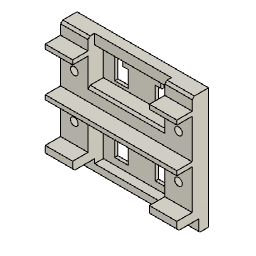
スタンドカップラー v1 (Autodesk Fusion 360 design; units mm, degrees)
Autodesk Fusion 360 part; units mm, degrees
note: some values were not read from the file. Chosen so that the rebuilt part matches the saved one: which bodies a step acts on; which face or edge a step refers to. Set by a fixed rule: which sketch regions a step uses.
sketch "スケッチ1" plane through (0, 0, 0) normal (0, 1, 0) x (1, 0, 0)
  line L0 (12.35, 21.95) -> (-12.35, 21.95) construction
  line L1 (-12.35, 21.95) -> (-12.35, -21.95) construction
  line L2 (-12.35, -21.95) -> (12.35, -21.95) construction
  line L3 (12.35, -21.95) -> (12.35, 21.95) construction
  line L4 (12.35, 21.95) -> (-12.35, -21.95) construction
  line L5 (-12.35, 21.95) -> (12.35, -21.95) construction
  line L6 (12.35, -21.95) -> (8.65, -21.95)
  line L7 (8.65, -21.95) -> (8.65, -15.35)
  line L8 (8.65, -8.35) -> (12.35, -8.35)
  line L9 (12.35, -8.35) -> (12.35, -21.95)
  line L10 (12.35, -8.35) -> (6.15, -8.35)
  line L11 (6.15, -8.35) -> (6.15, -15.35)
  line L12 (6.15, -15.35) -> (8.65, -15.35)
  line L13 (12.35, -15.35) -> (12.35, -8.35)
  line L14 (12.35, 21.95) -> (12.35, 8.35)
  line L15 (12.35, 14.95) -> (12.35, 21.95)
  line L16 (8.65, 21.95) -> (12.35, 21.95)
  line L17 (12.35, 21.95) -> (6.15, 21.95)
  line L18 (12.35, 8.35) -> (8.65, 8.35)
  line L19 (8.65, 8.35) -> (8.65, 14.95)
  line L20 (6.15, 14.95) -> (8.65, 14.95)
  line L21 (6.15, 21.95) -> (6.15, 14.95)
  line L22 (0, 0) -> (0, -7)
  line L23 (-12.35, 21.95) -> (12.35, 21.95) construction
  line L24 (-12.35, -8.35) -> (-12.35, -21.95)
  line L25 (-6.15, -15.35) -> (-8.65, -15.35)
  line L26 (-12.35, -21.95) -> (-8.65, -21.95)
  line L27 (-8.65, -21.95) -> (-8.65, -15.35)
  line L28 (-12.35, 21.95) -> (-6.15, 21.95)
  line L29 (-12.35, 21.95) -> (12.35, -21.95) construction
  line L30 (-12.35, -21.95) -> (-12.35, 21.95) construction
  line L31 (-8.65, 21.95) -> (-12.35, 21.95)
  line L32 (-8.65, 8.35) -> (-8.65, 14.95)
  line L33 (12.35, 21.95) -> (-12.35, -21.95) construction
  line L34 (12.35, -21.95) -> (-12.35, -21.95) construction
  line L35 (-12.35, 8.35) -> (-8.65, 8.35)
  line L36 (-6.15, 21.95) -> (-6.15, 14.95)
  line L37 (-8.65, -8.35) -> (-12.35, -8.35)
  line L38 (-12.35, -15.35) -> (-12.35, -8.35)
  line L39 (-6.15, 14.95) -> (-8.65, 14.95)
  line L40 (-6.15, -8.35) -> (-6.15, -15.35)
  line L41 (-12.35, 21.95) -> (-12.35, 8.35)
  line L42 (-12.35, -8.35) -> (-6.15, -8.35)
  line L43 (-12.35, 14.95) -> (-12.35, 21.95)
  line L44 (22.5, 32.5) -> (-22.5, 32.5)
  line L45 (-22.5, 32.5) -> (-22.5, -32.5)
  line L46 (-22.5, -32.5) -> (22.5, -32.5)
  line L47 (22.5, -32.5) -> (22.5, 32.5)
  line L48 (22.5, 32.5) -> (-22.5, -32.5) construction
  line L49 (-22.5, 32.5) -> (22.5, -32.5) construction
  dimension "d1" = 24.7
  dimension "d2" = 43.9
  dimension "d3" = 3.7
  dimension "d4" = 13.6
  dimension "d5" = 6.2
  dimension "d6" = 7
  dimension "d7" = 3.7
  dimension "d8" = 13.6
  dimension "d9" = 6.2
  dimension "d10" = 7
  dimension "d11" = 45
  dimension "d12" = 65
  constraint horizontal L0
  constraint perpendicular L0 L1
  constraint parallel L0 L2
  constraint parallel L1 L3
  constraint coincident L4 L22.start
  constraint coincident L5 L22.start
  constraint coincident L22.start origin
  constraint horizontal L6
  constraint vertical L7
  constraint horizontal L8
  constraint vertical L9
  constraint horizontal L10
  constraint vertical L11
  constraint horizontal L12
  constraint vertical L13
  constraint horizontal L18
  constraint vertical L19
  constraint horizontal L16
  constraint vertical L14
  constraint horizontal L17
  constraint vertical L21
  constraint horizontal L20
  constraint vertical L15
  constraint vertical L22
  constraint symmetric L0.start L22 L0.end
  constraint symmetric L0.end L22 L0.start
  constraint symmetric L1.end L22 L2.end
  constraint symmetric L2.end L22 L1.end
  constraint symmetric L6.end L22 L26.end
  constraint symmetric L8.start L22 L37.start
  constraint symmetric L8.end L22 L24.start
  constraint symmetric L10.end L22 L40.start
  constraint symmetric L11.end L22 L25.start
  constraint symmetric L13.start L22 L38.start
  constraint symmetric L7.end L22 L25.end
  constraint symmetric L19.end L22 L32.end
  constraint symmetric L17.end L22 L28.end
  constraint symmetric L15.start L22 L43.start
  constraint symmetric L20.start L22 L36.end
  constraint symmetric L18.end L22 L32.start
  constraint symmetric L14.end L22 L35.start
  constraint symmetric L16.start L22 L31.start
  constraint horizontal L44
  constraint perpendicular L44 L45
  constraint parallel L44 L46
  constraint parallel L45 L47
  constraint coincident L48 L22.start
  constraint coincident L49 L22.start
  measures "d1" distance of L1.end L2.end
  measures "d2" distance of L0.end L1.end
  measures "d3" distance of L2.end L6.end
  measures "d4" distance of L2.end L8.end
  measures "d5" distance of L8.end L10.end
  measures "d6" distance of L8.end L13.start
  measures "d7" distance of L18.end L14.end
  measures "d8" distance of L0.start L14.end
  measures "d9" distance of L17.end L0.start
  measures "d10" distance of L15.start L0.start
  measures "d11" distance of L45.end L46.end
  measures "d12" distance of L44.end L45.end
extrude "押し出し1" add sketch "スケッチ1" along normal blind 1.46 makes body 1
sketch "スケッチ2" plane through (0, 0, 0) normal (0, -1, 0) x (1, 0, 0)
  line L0 (12.35, -8.35) -> (12.35, -21.95)
  line L1 (12.35, -21.95) -> (6.15, -21.95)
  line L2 (6.15, -21.95) -> (6.15, -14.95)
  line L3 (6.15, -14.95) -> (8.65, -14.95)
  line L4 (8.65, -14.95) -> (8.65, -8.35)
  line L5 (8.65, -8.35) -> (12.35, -8.35)
  line L6 (-12.35, 8.35) -> (-12.35, 21.95)
  line L7 (-12.35, 21.95) -> (-8.65, 21.95)
  line L8 (-8.65, 21.95) -> (-8.65, 15.35)
  line L9 (-8.65, 15.35) -> (-6.15, 15.35)
  line L10 (-6.15, 15.35) -> (-6.15, 8.35)
  line L11 (-6.15, 8.35) -> (-12.35, 8.35)
  line L12 (-12.35, -8.35) -> (-8.65, -8.35)
  line L13 (-8.65, -8.35) -> (-8.65, -14.95)
  line L14 (-8.65, -14.95) -> (-6.15, -14.95)
  line L15 (-6.15, -14.95) -> (-6.15, -21.95)
  line L16 (-6.15, -21.95) -> (-12.35, -21.95)
  line L17 (-12.35, -21.95) -> (-12.35, -8.35)
  line L18 (12.35, 21.95) -> (12.35, 8.35)
  line L19 (12.35, 8.35) -> (6.15, 8.35)
  line L20 (6.15, 8.35) -> (6.15, 15.35)
  line L21 (6.15, 15.35) -> (8.65, 15.35)
  line L22 (8.65, 15.35) -> (8.65, 21.95)
  line L23 (8.65, 21.95) -> (12.35, 21.95)
  line L24 (22.5, -32.5) -> (22.5, 32.5)
  line L25 (22.5, 32.5) -> (-22.5, 32.5)
  line L26 (-22.5, 32.5) -> (-22.5, -32.5)
  line L27 (-22.5, -32.5) -> (22.5, -32.5)
  line L28 (-8.65, 21.95) -> (22.5, 21.95)
  line L29 (-12.35, 21.95) -> (-22.5, 21.95)
  line L30 (-12.35, -8.35) -> (-22.5, -8.35)
  line L31 (-8.65, -8.35) -> (8.65, -8.35)
  line L32 (12.35, -8.35) -> (22.5, -8.35)
  line L33 (-22.5, 0) -> (22.5, 0)
  line L34 (-6.15, 15.35) -> (6.15, 15.35)
  line L35 (-6.15, -14.95) -> (6.15, -14.95)
  constraint coincident L7.end L8.start
  constraint coincident L24 L28.end
  constraint perpendicular L24 L28
  constraint coincident L6.end L7.start
  constraint coincident L26 L29.end
  constraint perpendicular L26 L29
  constraint coincident L12.start L17.end
  constraint coincident L26 L30.end
  constraint perpendicular L26 L30
  constraint coincident L12.end L13.start
  constraint coincident L4.end L5.start
  constraint coincident L0.start L5.end
  constraint coincident L24 L32.end
  constraint perpendicular L24 L32
  constraint midpoint L26 L33.start
  constraint perpendicular L26 L33
  constraint coincident L9.end L10.start
  constraint coincident L20.end L21.start
  constraint coincident L14.end L15.start
  constraint coincident L2.end L3.start
extrude "押し出し2" add sketch "スケッチ2" along normal blind 4 contours L5 L12 L24 L26 L30 L31 L32 L33 | L3 L4 L13 L14 L31 L35 | L7 L23 L24 L25 L26 L28 L29 | L8 L9 L21 L22 L28 L34 bodies 1
move_face "面を移動1" by (0, 0, 7) 1 faces at (-7.5, -1.3333, 0) on bodies 1
sketch "スケッチ3" plane through (0, 0, 0) normal (0, -1, 0) x (1, 0, 0)
  line L0 (6.15, -14.95) -> (-6.15, -14.95)
  line L1 (-6.15, -14.95) -> (-6.15, -21.95)
  line L2 (-6.15, -21.95) -> (-12.35, -21.95)
  line L3 (-12.35, -21.95) -> (-12.35, -8.35)
  line L4 (-12.35, -8.35) -> (-22.5, -8.35)
  line L5 (-22.5, -8.35) -> (-22.5, -32.5)
  line L6 (-22.5, -32.5) -> (22.5, -32.5)
  line L7 (22.5, -32.5) -> (22.5, -8.35)
  line L8 (22.5, -8.35) -> (12.35, -8.35)
  line L9 (12.35, -8.35) -> (12.35, -21.95)
  line L10 (12.35, -21.95) -> (6.15, -21.95)
  line L11 (6.15, -21.95) -> (6.15, -14.95)
  line L12 (-22.5, -24.9494) -> (22.5, -24.9494)
  constraint coincident L5 L12.start
  constraint coincident L7 L12.end
  constraint perpendicular L7 L12
extrude "押し出し3" add sketch "スケッチ3" along normal blind 4 contours L5 L6 L7 L12 bodies 1
split "分割1" by plane through (0, 0, 0) normal (0, -1, 0) bodies 1 makes body 2 at (2.8833, -4, 1.8833) makes body 3 at (-7.5, -4, -27.4663) makes body 4 at (2.8833, -4, 28.9833)
move_face "面を移動2" by (0, 0, 6.5) 1 faces at (2.05, -2.6667, 15.35) on bodies 4
delete_face "面を削除1" 3 faces at (8.65, -2.6667, 21.9167) (2.8833, -2.6667, 21.85) (-8.65, -2.6667, 21.9167) on bodies 4
delete_face "面を削除2" 3 faces at (8.65, -1.3333, -12.75) (2.05, -2.6667, -14.95) (-8.65, -1.3333, -12.75) on bodies 2
chamfer "面取り1" distance 0.5 angle 45 1 edges at (-7.4, 0, 15.35) on bodies 1
chamfer "面取り2" distance 0.5 angle 45 3 edges at (7.4, 0, 15.35) (-7.4, 0, -14.95) (7.4, 0, -14.95) on bodies 1
sketch "スケッチ4" plane through (0, -4, 0) normal (0, -1, 0) x (1, 0, 0)
  line L0 (-22.5, -8.35) -> (22.5, -8.35)
  line L1 (22.5, -8.35) -> (22.5, 7)
  line L2 (22.5, 7) -> (-22.5, 7)
  line L3 (-22.5, 7) -> (-22.5, -8.35)
  line L4 (30, 17) -> (-30, 17)
  line L5 (-30, 17) -> (-30, -17)
  line L6 (-30, -17) -> (30, -17)
  line L7 (30, -17) -> (30, 17)
  line L8 (30, 17) -> (-30, -17) construction
  line L9 (-30, 17) -> (30, -17) construction
  line L10 (17.5, -17.4093) -> (-17.5, -17.4093)
  line L11 (-17.5, -17.4093) -> (-17.5, 17.4093)
  line L12 (-17.5, 17.4093) -> (17.5, 17.4093)
  line L13 (17.5, 17.4093) -> (17.5, -17.4093)
  line L14 (17.5, -17.4093) -> (-17.5, 17.4093) construction
  line L15 (-17.5, -17.4093) -> (17.5, 17.4093) construction
  dimension "d21" = 60
  dimension "d22" = 34
  dimension "d23" = 35
  constraint horizontal L4
  constraint perpendicular L4 L5
  constraint parallel L4 L6
  constraint parallel L5 L7
  constraint coincident L8 origin
  constraint coincident L9 origin
  constraint horizontal L10
  constraint perpendicular L10 L11
  constraint parallel L10 L12
  constraint parallel L11 L13
  constraint coincident L14 origin
  constraint coincident L15 origin
  measures "d21" distance of L5.end L6.end
  measures "d22" distance of L4.end L5.end
  measures "d23" distance of L11.end L12.end
extrude "押し出し4" add sketch "スケッチ4" against normal blind 5.46 contours L0 L2 L3 L4 L5 L6 L11 | L0 L1 L2 L4 L6 L7 L13 bodies 1 2
move_face "面を移動3" by (0, -3, 0) 1 faces at (5.8333, -4, 1.8833) on bodies 1
move_face "面を移動4" by (0, 0, -15.5) 2 faces at (-23.3333, -4.6667, -17) (23.3333, -4.6667, -17) on bodies 1
move_face "面を移動5" by (0, 0, 15.5) 2 faces at (23.3333, -4.6667, 17) (-23.3333, -4.6667, 17) on bodies 1
sketch "スケッチ5" plane through (0, -7, 0) normal (0, -1, 0) x (1, 0, 0)
  line L0 (-17.5, -8.35) -> (17.5, -8.35)
  line L1 (17.5, -8.35) -> (17.5, -32.5)
  line L2 (17.5, -32.5) -> (30, -32.5)
  line L3 (30, -32.5) -> (30, 32.5)
  line L4 (30, 32.5) -> (17.5, 32.5)
  line L5 (17.5, 32.5) -> (17.5, 7)
  line L6 (17.5, 7) -> (-17.5, 7)
  line L7 (-17.5, 7) -> (-17.5, 32.5)
  line L8 (-17.5, 32.5) -> (-30, 32.5)
  line L9 (-30, 32.5) -> (-30, -32.5)
  line L10 (-30, -32.5) -> (-17.5, -32.5)
  line L11 (-17.5, -32.5) -> (-17.5, -8.35)
  line L12 (30, -1) -> (-30, -1)
  line L13 (-30, -1) -> (-30, 1)
  line L14 (-30, 1) -> (30, 1)
  line L15 (30, 1) -> (30, -1)
  line L16 (30, -1) -> (-30, 1) construction
  line L17 (-30, -1) -> (30, 1) construction
  dimension "d26" = 60
  dimension "d27" = 2
  constraint horizontal L12
  constraint perpendicular L12 L13
  constraint parallel L12 L14
  constraint parallel L13 L15
  constraint coincident L16 origin
  constraint coincident L17 origin
  measures "d26" distance of L13.end L14.end
  measures "d27" distance of L12.end L13.end
extrude "押し出し5" add sketch "スケッチ5" along normal blind 5 contours L3 L9 L12 L13 L14 L15 bodies 1
sketch "スケッチ6" plane through (0, -7, 0) normal (0, -1, 0) x (1, 0, 0)
  line L0 (-30, 1) -> (30, 1)
  line L1 (30, 1) -> (30, 32.5)
  line L2 (30, 32.5) -> (17.5, 32.5)
  line L3 (17.5, 32.5) -> (17.5, 7)
  line L4 (17.5, 7) -> (-17.5, 7)
  line L5 (-17.5, 7) -> (-17.5, 32.5)
  line L6 (-17.5, 32.5) -> (-30, 32.5)
  line L7 (-30, 32.5) -> (-30, 1)
  line L8 (-30, 1) -> (30, 1)
  line L9 (30, 1) -> (30, 19)
  line L10 (30, 19) -> (-30, 19)
  line L11 (-30, 19) -> (-30, 1)
  line L12 (-17.5, 7) -> (-17.5, 1)
  line L13 (17.5, 7) -> (17.5, 1)
  line L14 (-6, 0) -> (5, 0)
  line L15 (30, -19) -> (-30, -19)
  line L16 (-30, -19) -> (-30, -1)
  line L17 (-17.5, -7) -> (-17.5, -32.5)
  line L18 (-17.5, -7) -> (-17.5, -1)
  line L19 (17.5, -32.5) -> (17.5, -7)
  line L20 (17.5, -7) -> (17.5, -1)
  line L21 (30, -1) -> (30, -19)
  line L22 (-30, 19) -> (30, 19)
  line L23 (30, 19) -> (30, 21)
  line L24 (30, 21) -> (-30, 21)
  line L25 (-30, 21) -> (-30, 19)
  line L26 (-30, -19) -> (30, -19)
  line L27 (30, -19) -> (30, -21)
  line L28 (30, -21) -> (-30, -21)
  line L29 (-30, -21) -> (-30, -19)
  line L30 (-30, 19) -> (-17.5, 1)
  line L31 (-17.5, 19) -> (-30, 1)
  circle A0 centre (-23.75, 10) radius 1.75
  line L32 (0, 0) -> (0, 4)
  circle A1 centre (23.75, 10) radius 1.75
  circle A2 centre (-23.75, -10) radius 1.75
  circle A3 centre (23.75, -10) radius 1.75
  dimension "d30" = 60
  dimension "d31" = 18
  dimension "d32" = 60
  dimension "d33" = 2
  dimension "d34" = 2
  dimension "d35" = 3.5
  constraint horizontal L8
  constraint vertical L9
  constraint horizontal L10
  constraint vertical L11
  constraint coincident L0.start L7.end
  constraint coincident L4.end L5.start
  constraint perpendicular L4 L12
  constraint coincident L3.end L4.start
  constraint coincident L8 L13.end
  constraint perpendicular L8 L13
  constraint perpendicular L13 L14
  constraint symmetric L2.end L14 L19.start
  constraint symmetric L3.end L14 L19.end
  constraint symmetric L4.end L14 L17.start
  constraint symmetric L5.end L14 L17.end
  constraint symmetric L0.start L14 L16.end
  constraint symmetric L0.end L14 L21.start
  constraint symmetric L9.end L14 L15.start
  constraint symmetric L10.end L14 L15.end
  constraint symmetric L12.end L14 L18.end
  constraint symmetric L13.end L14 L20.end
  constraint horizontal L22
  constraint vertical L23
  constraint horizontal L24
  constraint vertical L25
  constraint horizontal L26
  constraint vertical L27
  constraint horizontal L28
  constraint vertical L29
  constraint coincident L10 L31.start
  constraint coincident L5 L31.start
  constraint midpoint L30 A0.centre
  constraint coincident L32.start origin
  constraint perpendicular L8 L32
  constraint symmetric A0 L32 A1
  constraint symmetric L14 A0 A2
  constraint symmetric L14 A1 A3
  measures "d30" distance of L0.start L0.end
  measures "d31" distance of L0.start L10.end
  measures "d32" distance of L10.end L9.end
  measures "d33" distance of L10.end L24.end
  measures "d34" distance of L15.end L28.end
  measures "d35" diameter of A0
extrude "押し出し6" add sketch "スケッチ6" along normal blind 5 contours L5 L7 L10 L22 L24 L25 | L1 L3 L10 L22 L23 L24 | L15 L19 L26 L27 L28 | L15 L17 L26 L28 L29 bodies 1
extrude "押し出し7" cut sketch "スケッチ6" against normal blind 29 contours L30 L31 A0 | L30 L31 A0 | L30 L31 A0 | L30 L31 A0 | A1 | A2 | A3 bodies 1
combine "結合1" operation add target body 1 tool bodies 3 4
move_face "面を移動6" by (0, 0, -6) 1 faces at (25.8333, -3.18, 32.5) on bodies 1
move_face "面を移動7" by (0, 0, 4) 1 faces at (25.8333, -3.18, -32.5) on bodies 1
move_face "面を移動8" by (0, 3, 0) 2 faces at (-21.6667, -7, -23.5) (21.6667, -7, -23.5) on bodies 1
chamfer "面取り3" distance 0.5 angle 45 1 edges at (0, -4, -28.5) on bodies 1
chamfer "面取り4" distance 1 angle 45 4 edges at (0, 1.46, -28.5) (-30, 1.46, -1) (30, 1.46, -1) (0, 1.46, 26.5) on bodies 1
chamfer "面取り5" distance 1 angle 45 4 edges at (0, -7, 7) (-23.75, -7, 26.5) (23.75, -7, 26.5) (0, -7, -8.35) on bodies 1
move_face "面を移動9" by (0, -2, 0) 5 faces at (-25.8333, -12, -19.6667) (25.8333, -12, -20.3333) (-10, -12, -0.3333) (-21.6667, -12, 20.3333) (21.6667, -12, 19.6667) on bodies 1
move_face "面を移動10" by (0, 0, -2) 2 faces at (-21.6667, -7.3333, -21) (21.6667, -8.3333, -21) on bodies 1
chamfer "面取り6" distance 1 angle 45 2 edges at (-23.75, -14, -23) (23.75, -14, -23) on bodies 1
